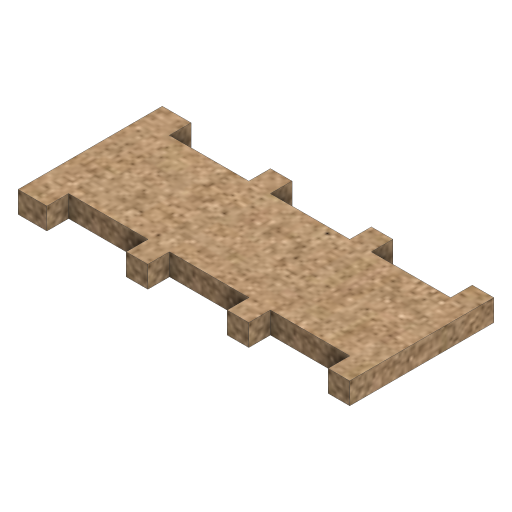
# Autodesk Inventor part: side_wall_short
Saved by Autodesk Inventor 2024 (Build 280153000, 153)
## iProperties
Created: 2024-06-06
Material: MDF Medium Density Fiberboard
Document SubType Name: Modeling
Designer: USER
Density: 0.8 g/cm^3
Appearance: Cardboard - Corrugated
Mass: 1.7328 g
Surface Area: 19.48 cm^2
Volume: 2.166 cm^3
Author: 第26組
Title: side_wall_short
Autodesk Inventor part; units mm, degrees
ref_plane "YZ Plane" through (0, 0, 0) normal (1, 0, 0) x (0, 1, 0)
ref_plane "XZ Plane" through (0, 0, 0) normal (0, 1, 0) x (-1, 0, 0)
ref_plane "XY Plane" through (0, 0, 0) normal (0, 0, 1) x (1, 0, 0)
sketch "草圖2" plane through (0, 0, 0) normal (0, 1, 0) x (-1, 0, 0)
  line L0 (0, 0) -> (31, 0)
  line L1 (31, 0) -> (31, -14)
  line L2 (31, -14) -> (0, -14)
  line L3 (0, -14) -> (0, 0)
  line L4 (31, -14) -> (28, -14)
  line L5 (28, -14) -> (28, -17)
  line L6 (28, -17) -> (31, -17)
  line L7 (31, -17) -> (31, -14)
  line L8 (31, -7) -> (0, -7)
  line L9 (15.5, -14) -> (15.5, 0)
  line L10 (28, 0) -> (28, 3)
  line L11 (28, 3) -> (31, 3)
  line L12 (31, 3) -> (31, 0)
  line L13 (3, -14) -> (3, -17)
  line L14 (3, -17) -> (0, -17)
  line L15 (0, -17) -> (0, -14)
  line L16 (3, 0) -> (3, 3)
  line L17 (3, 3) -> (0, 3)
  line L18 (0, 3) -> (0, 0)
  line L19 (17, -14) -> (14, -14)
  line L20 (14, -14) -> (14, -17)
  line L21 (14, -17) -> (17, -17)
  line L22 (17, -17) -> (17, -14)
  line L23 (14, 0) -> (14, 3)
  line L24 (14, 3) -> (17, 3)
  line L25 (17, 3) -> (17, 0)
  line L26 (31, 0) -> (46, 0)
  line L27 (46, 0) -> (46, -14)
  line L28 (46, -14) -> (31, -14)
  line L29 (31, -14) -> (31, 0)
  line L30 (45, -14) -> (42, -14)
  line L31 (42, -14) -> (42, -17)
  line L32 (42, 0) -> (42, 3)
  line L33 (42, -17) -> (46, -17)
  line L34 (46, -14) -> (46, -17)
  line L35 (42, 3) -> (46, 3)
  line L36 (46, 0) -> (46, 3)
  point P0 (44, 3)
  dimension "d9" = 31
  dimension "d10" = 14
  dimension "d11" = 3
  dimension "d12" = 3
  dimension "d13" = 3
  dimension "d14" = 3
  dimension "d18" = 11
  dimension "d21" = 14
  dimension "d22" = 46
  dimension "d23" = 20
  constraints: 74 end point, 16 symmetric about line, 8 parallel, 6 horizontal, 6 midpoint, 6 perpendicular, 1 horizontal alignment
  measures "d9" distance of L1.end L2.end
  measures "d10" distance of L2.end L0.start
  measures "d11" distance of L5.end L6.end
  measures "d12" distance of L4.end L5.end
  measures "d13" distance of L19.end L20.end
  measures "d14" distance of L20.end L21.end
  measures "d18" distance of L1.end L30.end
  measures "d21" distance of L26.end L27.end
  measures "d22" distance between parallel lines of L3 L27
  measures "d23" distance from line of point (44, 3) L33
extrude "擠出2" add sketch "草圖2" along normal blind 3
